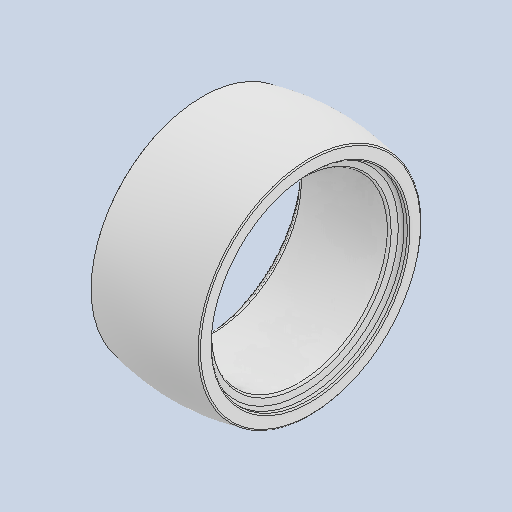
# Autodesk Inventor part: ToePalm
Saved by Autodesk Inventor 2022.2 (Build 262287030, 287C)
## iProperties
Created: 2021-12-28
Part Number: ToePalm
Material: Generic
Document SubType Name: Modeling
Designer: Jochen
Density: 1 g/cm^3
Appearance: Default
Author: Jochen
Autodesk Inventor part; units mm, degrees
ref_plane "YZ Plane" through (0, 0, 0) normal (1, 0, 0) x (0, 1, 0)
ref_plane "XZ Plane" through (0, 0, 0) normal (0, 1, 0) x (-1, 0, 0)
ref_plane "XY Plane" through (0, 0, 0) normal (0, 0, 1) x (1, 0, 0)
derived "Toe.ipt"
sketch "ToeSketch" plane through (0, 0, 0) normal (0, 0, 1) x (1, 0, 0)
  line L0 (-16.2724, 0) -> (16.3247, 0) construction
  line L1 (0, -21.6048) -> (0, 20.9058) construction
  line L2 (-8.25, 12.3131) -> (-8.25, 11.2)
  line L3 (8.25, 12.4247) -> (8.25, 11.2)
  line L4 (0.75, 0.7) -> (0.75, 9)
  line L5 (0.75, 0.7) -> (-0.75, 0.7)
  line L6 (-0.75, 0.7) -> (-0.75, 9)
  line L7 (-8.05, 11) -> (-7.7872, 11)
  arc A0 (-2.8714, 11.0781) -> (-7.6286, 11.0781) centre (-5.25, 9.25) ccw
  arc A1 (7.6286, 11.0781) -> (2.8714, 11.0781) centre (5.25, 9.25) ccw
  line L8 (7.7872, 11) -> (8.05, 11)
  arc A2 (8.05, 11) -> (8.25, 11.2) centre (8.05, 11.2) ccw
  arc A3 (8.25, 12.4247) -> (7.9777, 12.8037) centre (7.85, 12.4247) ccw
  arc A4 (-6.4776, 13.2808) -> (-8.25, 12.3131) centre (-7.2869, 12.6561) ccw
  arc A5 (-8.25, 11.2) -> (-8.05, 11) centre (-8.05, 11.2) ccw
  arc A6 (-7.7872, 11) -> (-7.6286, 11.0781) centre (-7.7872, 11.2) ccw
  arc A7 (7.6286, 11.0781) -> (7.7872, 11) centre (7.7872, 11.2) ccw
  arc A8 (6.4776, 13.2808) -> (-6.4776, 13.2808) centre (0, -15.5318) ccw
  circle A9 centre (-5.25, 9.25) radius 3 construction
  circle A10 centre (5.25, 9.25) radius 3 construction
  line L9 (5.8717, 12.1849) -> (6.1204, 13.3588) construction
  line L10 (8.25, 12.4247) -> (8.25, 14.35)
  line L11 (7.85, 14.75) -> (7.55, 14.75)
  line L12 (7.0939, 14.3486) -> (7.0939, 14.1843)
  line L13 (-8.25, 12.3131) -> (-8.25, 14.35)
  line L14 (-7.85, 14.75) -> (-7.55, 14.75)
  arc A11 (8.25, 14.35) -> (7.85, 14.75) centre (7.85, 14.35) ccw
  arc A12 (7.55, 14.75) -> (7.1609, 14.4429) centre (7.55, 14.35) ccw
  arc A13 (-7.1609, 14.4429) -> (-7.55, 14.75) centre (-7.55, 14.35) ccw
  arc A14 (-7.85, 14.75) -> (-8.25, 14.35) centre (-7.85, 14.35) ccw
  arc A15 (-6.9544, 13.5782) -> (-6.4776, 13.2808) centre (-6.5653, 13.6711) ccw
  arc A16 (6.4776, 13.2808) -> (6.9544, 13.5782) centre (6.5653, 13.6711) ccw
  line L15 (-7.1609, 14.4429) -> (-6.9544, 13.5782)
  line L16 (6.9544, 13.5782) -> (7.1609, 14.4429)
  line L17 (0.75, 9) -> (1.75, 9)
  line L18 (-0.75, 9) -> (-1.75, 9)
  arc A17 (2.7128, 11) -> (2.8714, 11.0781) centre (2.7128, 11.2) ccw
  line L19 (2.7128, 11) -> (1.75, 11)
  line L20 (1.75, 11) -> (1.75, 9)
  line L21 (-1.75, 9) -> (-1.75, 11)
  line L22 (-1.75, 11) -> (-2.7128, 11)
  arc A18 (-2.8714, 11.0781) -> (-2.7128, 11) centre (-2.7128, 11.2) ccw
  line L23 (8.05, 11) -> (8.6386, 11)
  line L24 (8.6386, 11) -> (8.6386, 9.9)
  line L25 (9.0386, 9.5) -> (11.15, 9.5)
  arc A19 (11.15, 9.5) -> (11.4713, 10.1383) centre (11.15, 9.9) ccw
  arc A20 (8.6386, 9.9) -> (9.0386, 9.5) centre (9.0386, 9.9) ccw
  line L26 (-8.05, 11) -> (-8.6386, 11)
  line L27 (-8.6386, 11) -> (-8.6386, 9.9)
  line L28 (-9.0386, 9.5) -> (-11, 9.5)
  line L29 (-11.3819, 10.2587) -> (-8.1713, 14.5883)
  arc A21 (-9.0386, 9.5) -> (-8.6386, 9.9) centre (-9.0386, 9.9) ccw
  arc A22 (-11.3819, 10.2587) -> (-11, 9.5) centre (-11, 9.9755) ccw
  line L30 (11.4713, 10.1383) -> (8.1713, 14.5883)
  line L31 (-1.75, 11) -> (-1.25, 11)
  line L32 (-0.75, 10.5) -> (-0.75, 9)
  line L33 (0.75, 9) -> (0.75, 10.5)
  line L34 (1.75, 11) -> (1.25, 11)
  arc A23 (-0.75, 10.5) -> (-1.25, 11) centre (-1.25, 10.5) ccw
  arc A24 (1.25, 11) -> (0.75, 10.5) centre (1.25, 10.5) ccw
  line L35 (-7.6286, 11.0781) -> (-8.7214, 9.6562)
  line L36 (7.6286, 11.0781) -> (8.7214, 9.6562)
  point P0 (0, 0)
  point P1 (-8.25, 10.6859)
  point P2 (8.25, 11)
  point P3 (-7.6867, 11)
  point P4 (2.8133, 11)
  point P5 (0, 14)
  point P6 (7.6867, 11)
  point P7 (0.75, 11)
  point P8 (2.4071, 10.208)
  point P9 (8.6386, 9.5)
  point P10 (8.1328, 14.6328)
  point P11 (-0.75, 11)
  point P12 (11.55, 9.9)
  point P13 (2.2314, 11)
sketch "Sketch2" plane through (0, 0, 0) normal (0, 0, 1) x (1, 0, 0)
  line L0 (0, -25.14) -> (0, 25.015) construction
  line L1 (-16.2724, 0) -> (16.3247, 0) construction
  arc A0 (8.0985, 16.8527) -> (-8.0985, 16.8527) centre (0, -15.5318) ccw
  arc A1 (6.4776, 13.2808) -> (-6.4776, 13.2808) centre (0, -15.5318) ccw construction
  line L2 (-8.25, 12.3131) -> (-8.25, 11.2) construction
  arc A2 (8.25, 12.4247) -> (7.9777, 12.8037) centre (7.85, 12.4247) ccw construction
  line L3 (8.25, 12.4247) -> (8.25, 11.2) construction
  arc A3 (6.4995, 13.3784) -> (-6.4995, 13.3784) centre (0, -15.5318) ccw
  line L4 (-8.05, 11) -> (-7.7872, 11) construction
  arc A4 (-8.25, 11.2) -> (-8.05, 11) centre (-8.05, 11.2) ccw construction
  line L5 (7.7872, 11) -> (8.05, 11) construction
  arc A5 (8.05, 11) -> (8.25, 11.2) centre (8.05, 11.2) ccw construction
  arc A6 (-6.8571, 13.6014) -> (-6.4995, 13.3784) centre (-6.5653, 13.6711) ccw
  arc A7 (6.4995, 13.3784) -> (6.8571, 13.6014) centre (6.5653, 13.6711) ccw
  line L6 (7.55, 14.85) -> (8.05, 14.85)
  arc A8 (8.05, 14.85) -> (8.25, 15.05) centre (8.05, 15.05) ccw
  line L7 (-7.55, 14.85) -> (-8.05, 14.85)
  arc A9 (-8.25, 15.05) -> (-8.05, 14.85) centre (-8.05, 15.05) ccw
  line L8 (8.25, 14.35) -> (8.25, 15.05) construction
  line L9 (8.25, 12.4247) -> (8.25, 14.35) construction
  arc A10 (-7.0637, 14.4662) -> (-7.55, 14.85) centre (-7.55, 14.35) ccw
  line L10 (-7.0637, 14.4662) -> (-6.8571, 13.6014)
  line L11 (-7.1609, 14.4429) -> (-6.9544, 13.5782) construction
  line L12 (6.8571, 13.6014) -> (7.0637, 14.4662)
  arc A11 (7.55, 14.85) -> (7.0637, 14.4662) centre (7.55, 14.35) ccw
  line L13 (8.25, 15.05) -> (8.25, 16.6587)
  arc A12 (8.25, 16.6587) -> (8.0985, 16.8527) centre (8.05, 16.6587) ccw
  line L14 (-8.25, 15.05) -> (-8.25, 16.6587)
  arc A13 (-8.0985, 16.8527) -> (-8.25, 16.6587) centre (-8.05, 16.6587) ccw
  point P0 (0, 0)
  point P1 (0, 17.85)
  point P2 (7.55, 14.35)
  dimension "d3" = 3.75
  dimension "d6" = 0.1
  dimension "d19" = 0.2
  constraints: 21 point on circle, 14 end point, 14 tangent, 10 centre point, 2 coincident, 2 collinear, 2 horizontal, 2 vertical, 1 concentric, 1 equal radius, 1 parallel, 8 other
  measures "d3" radial gap between concentric circles of A0 A3
  measures "d19" radius of A8
revolve "Revolution1" add sketch "Sketch2" angle 360 about axis through (-10, 0, 0) along (1, 0, 0)
body "Solid1"
